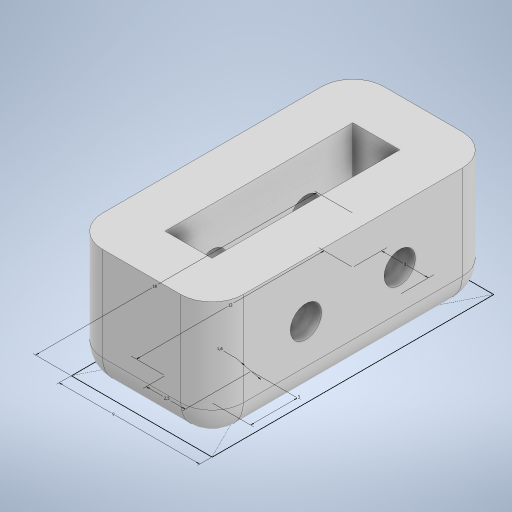
# Autodesk Inventor part: 3mm
Saved by Autodesk Inventor 2024 (Build 280153000, 153)
## iProperties
Created: 2023-12-03
Part Number: 3mm
Material: Všeobecné
Document SubType Name: Modeling
Designer: Roman Suk
Density: 1 g/cm^3
Appearance: Výchozí
MASSSFP: 400 g
SFP: 4HR
Author: Roman Suk
## iProperties of the stored document Part1_3DPrint.ipt
Created: 2023-12-03
Part Number: Part1_3DPrint
Material: Generic
Document SubType Name: Modeling
Designer: Roman Suk
Density: 1 g/cm^3
Appearance: Default
Author: Roman Suk
Autodesk Inventor part; units mm, degrees
ref_plane "YZ Plane" through (0, 0, 0) normal (1, 0, 0) x (0, 1, 0)
ref_plane "XZ Plane" through (0, 0, 0) normal (0, 1, 0) x (-1, 0, 0)
ref_plane "XY Plane" through (0, 0, 0) normal (0, 0, 1) x (1, 0, 0)
sketch "Sketch2" plane through (0, 0, 0) normal (0, 1, 0) x (-1, 0, 0)
  line L0 (-1.5, 6) -> (1.5, 6)
  line L1 (1.5, 6) -> (1.5, -6)
  line L2 (1.5, -6) -> (-1.5, -6)
  line L3 (-1.5, -6) -> (-1.5, 6)
  line L4 (-1.5, 6) -> (1.5, -6) construction
  line L5 (1.5, 6) -> (-1.5, -6) construction
  line L6 (1.5, 0) -> (-1.5, 0)
  circle A0 centre (-1, 3) radius 0.8
  circle A1 centre (-1, -3) radius 0.8
  line L7 (-4.5, -9) -> (4.5, -9)
  line L8 (4.5, -9) -> (4.5, 9)
  line L9 (4.5, 9) -> (-4.5, 9)
  line L10 (-4.5, 9) -> (-4.5, -9)
  line L11 (-4.5, -9) -> (4.5, 9) construction
  line L12 (4.5, -9) -> (-4.5, 9) construction
  point P0 (0, 0)
  dimension "d2" = 3
  dimension "d3" = 12
  dimension "d4" = 1.6
  dimension "d5" = 2.5
  dimension "d6" = 3
  dimension "d7" = 9
  dimension "d8" = 18
  constraints: 26 end point, 6 midpoint, 4 parallel, 2 centre point, 2 horizontal, 2 perpendicular, 1 symmetric about line, 1 other
  measures "d2" distance of L1.end L2.end
  measures "d3" distance of L0.end L1.end
  measures "d4" diameter of A0
  measures "d5" distance from line of L1 A0.centre
  measures "d6" distance from line of L0 A0.centre
  measures "d7" distance of L9.end L8.end
  measures "d8" distance of L8.end L7.end
extrude "Extrusion2" add sketch "Sketch2" along normal blind 2 contours L0 L1 L6 L3 A0 | A0 L3 | L1 L2 L3 A1 L6 | A1 L3 picked at (-1.0814, 3.2162) picked at (-1.0814, -2.7838)
extrude "Extrusion3" add sketch "Sketch2" along normal blind 8 contours L3 A0 | L3 A1 | L10 L9 L8 L7 picked at (-1.5421, 2.834) picked at (-1.5421, -3.166)
fillet "Fillet1" radius 2 8 edges at (-4.5, 0, 0) (0, 0, -9) (4.5, 0, 0) (0, 0, 9) (-4.5, 4, -9) (-4.5, 4, 9) (4.5, 4, 9) (4.5, 4, -9)
sketch "Sketch4" plane through (-4.5, 0, -9) normal (-1, 0, 0) x (0, 0, 1)
  line L0 (0, 0) -> (18, 0) construction
  line L1 (18, 0) -> (18, 8) construction
  line L2 (0, 0) -> (18, 0) construction
  line L3 (18, 0) -> (18, 2) construction
  line L4 (18, 2) -> (0, 2) construction
  line L5 (0, 2) -> (0, 0) construction
  line L6 (9, 0) -> (9, 8)
  line L7 (0, 8) -> (18, 8) construction
  circle A0 centre (6, 4.5) radius 1
  circle A1 centre (12, 4.5) radius 1
  dimension "d13" = 2
  dimension "d15" = 2
  dimension "d16" = 6
  dimension "d17" = 2.5
  constraints: 10 end point, 2 centre point, 2 parallel, 1 horizontal, 1 midpoint, 1 perpendicular, 1 point on line, 1 symmetric about line, 1 other
  measures "d13" distance of L3.end L2.end
  measures "d15" diameter of A0
  measures "d16" diameter of A0.centre L6
  measures "d17" distance from line of L4 A0.centre
extrude "Extrusion4" cut sketch "Sketch4" against normal through all
body "Solid2"
